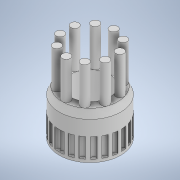
# Autodesk Inventor part: piece_roue_test_6
Saved by Autodesk Inventor 2020.1 (Build 241239000, 239)
## iProperties
Created: 2019-07-25
Part Number: piece_roue_test_6
Material: Générique
Document SubType Name: Modeling
Designer: marlo
Density: 1 g/cm^3
Appearance: Par défaut
Author: marlo
Autodesk Inventor part; units mm, degrees
ref_plane "YZ Plane" through (0, 0, 0) normal (1, 0, 0) x (0, 1, 0)
ref_plane "XZ Plane" through (0, 0, 0) normal (0, 1, 0) x (-1, 0, 0)
ref_plane "XY Plane" through (0, 0, 0) normal (0, 0, 1) x (1, 0, 0)
sketch "Esquisse2" plane through (0, 0, 0) normal (0, 1, 0) x (-1, 0, 0)
  circle A0 centre (0, 0) radius 18.5
  circle A1 centre (0, 0) radius 13.1
  dimension "d0" = 37
  dimension "d1" = 26.2
  constraints: 2 centre point, 2 coincident
  measures "d0" diameter of A0
  measures "d1" diameter of A1
extrude "Extrusion1" add sketch "Esquisse2" against normal blind 13
sketch "Esquisse3" plane through (0, 0, 0) normal (0, 1, 0) x (1, 0, 0)
  circle A0 centre (0, -15.8) radius 2.7
  line L0 (-22, 0) -> (25, 0) construction
  line L1 (-20, -18.5) -> (14, -18.5) construction
  circle A1 centre (0, 0) radius 18.5 construction
  circle A2 centre (-15.0267, 4.8825) radius 2.7
  line L2 (0, -15.8) -> (0, 0) construction
  line L3 (-15.0267, 4.8825) -> (0, 0) construction
  circle A3 centre (-15.0267, -4.8825) radius 2.7
  line L4 (0, 0) -> (-15.0267, -4.8825) construction
  line L5 (-15.0267, -4.8825) -> (-15.0267, 4.8825) construction
  line L6 (0, -31) -> (0, 24) construction
  line L7 (-15.0267, -4.8825) -> (-15.0267, -7.5825) construction
  line L8 (-15.0267, 4.8825) -> (-16.4693, 2.6002) construction
  line L9 (0, -15.8) -> (-2.3383, -17.15) construction
  circle A4 centre (-9.287, 12.7825) radius 2.7
  line L10 (0, 0) -> (-9.287, 12.7825) construction
  line L11 (-9.287, 12.7825) -> (-15.0267, 4.8825) construction
  line L12 (-9.287, 12.7825) -> (-7.7, 14.9668) construction
  circle A5 centre (-9.287, -12.7825) radius 2.7
  line L13 (-9.287, -12.7825) -> (0, 0) construction
  line L14 (-9.287, -12.7825) -> (0, -15.8) construction
  line L15 (-9.287, -12.7825) -> (-11.2119, -10.8891) construction
  line L16 (-9.287, -12.7825) -> (-15.0267, -4.8825) construction
  circle A6 centre (0, 15.8) radius 2.7
  line L17 (0, 15.8) -> (-1.5986, 17.9759) construction
  line L18 (0, 15.8) -> (0, 0) construction
  line L19 (0, 15.8) -> (-9.287, 12.7825) construction
  circle A7 centre (15.0267, 4.8825) radius 2.7
  circle A8 centre (15.0267, -4.8825) radius 2.7
  circle A9 centre (9.287, 12.7825) radius 2.7
  circle A10 centre (9.287, -12.7825) radius 2.7
  dimension "d4" = 5.4
  constraints: 40 end point, 14 equal length, 4 centre point, 4 symmetric about line, 3 horizontal, 3 point on line, 3 vertical, 1 coincident, 1 tangent, 1 vertical alignment, 21 other
extrude "Extrusion2" add sketch "Esquisse3" along normal blind 25
sketch "Esquisse4" plane through (0, -13, 0) normal (0, -1, 0) x (1, 0, 0)
  circle A0 centre (0, 0) radius 20.5
  circle A1 centre (0, 0) radius 13.1 projected
  circle A2 centre (0, 0) radius 18.5 projected
  circle A3 centre (0, 0) radius 13.1
  dimension "d9" = 2
  constraints: 2 centre point, 2 concentric, 1 coincident
  measures "d9" radial gap between concentric circles of A2 A0
extrude "Extrusion3" add sketch "Esquisse4" along normal blind 15 contours A0 | A2
sketch "Esquisse6" plane through (0, -13, 0) normal (0, 1, 0) x (1, 0, 0)
  line L0 (-3.2, -20.2487) -> (-3.1052, -19.6487)
  line L1 (0, -20.5) -> (0, -19.8926)
  arc A0 (0, -19.8926) -> (-3.1052, -19.6487) centre (-1.5707, -20.0012) ccw
  arc A1 (-3.2, -20.2487) -> (0, -20.5) centre (0, 0) ccw
  circle A2 centre (0, 0) radius 20.5 projected
  line L2 (0, 0) -> (-5.8325, -27.1444)
  line L3 (-5.4, -19.776) -> (-5.24, -19.19)
  line L4 (-8.4208, -18.6906) -> (-8.1713, -18.1368)
  arc A3 (-5.24, -19.19) -> (-8.1713, -18.1368) centre (-6.7838, -18.8811) ccw
  arc A4 (-8.4208, -18.6906) -> (-5.4, -19.776) centre (0, 0) ccw
  line L5 (0, 0) -> (0, -49) construction
  line L6 (-5.4, -19.776) -> (-3.2, -20.2487) construction
  line L7 (0, 0) -> (-12.1264, -23.3948)
  line L8 (-14.7012, -14.2872) -> (-14.2656, -13.8638)
  line L9 (-16.7512, -11.8172) -> (-16.2549, -11.4671)
  arc A5 (-14.2656, -13.8638) -> (-16.2549, -11.4671) centre (-15.4382, -12.8132) ccw
  arc A6 (-16.7512, -11.8172) -> (-14.7012, -14.2872) centre (0, 0) ccw
  line L10 (-13.0468, -15.8124) -> (-12.6602, -15.3438)
  line L11 (-10.4186, -17.6551) -> (-10.1099, -17.132)
  arc A7 (-10.1099, -17.132) -> (-12.6602, -15.3438) centre (-11.5178, -16.4273) ccw
  arc A8 (-13.0468, -15.8124) -> (-10.4186, -17.6551) centre (0, 0) ccw
  line L12 (-10.4186, -17.6551) -> (-8.4208, -18.6906) construction
  line L13 (0, 0) -> (-31.7535, -19.8843)
  line L14 (-19.6137, 5.9626) -> (-19.0325, 5.7859)
  line L15 (-18.4425, 8.9512) -> (-17.896, 8.6859)
  arc A9 (-19.0325, 5.7859) -> (-17.896, 8.6859) centre (-18.6796, 7.3203) ccw
  arc A10 (-18.4425, 8.9512) -> (-19.6137, 5.9626) centre (0, 0) ccw
  line L16 (-20.149, 3.777) -> (-19.552, 3.6651)
  line L17 (-20.4916, 0.5855) -> (-19.8844, 0.5681)
  arc A11 (-19.8844, 0.5681) -> (-19.552, 3.6651) centre (-19.9482, 2.1413) ccw
  arc A12 (-20.149, 3.777) -> (-20.4916, 0.5855) centre (0, 0) ccw
  line L18 (-20.149, 3.777) -> (-19.6137, 5.9626) construction
  line L19 (-19.2724, -6.9874) -> (-18.7014, -6.7803)
  line L20 (-17.9455, -9.9101) -> (-17.4137, -9.6164)
  line L21 (-19.9222, -4.833) -> (-19.3318, -4.6898)
  arc A13 (-17.4137, -9.6164) -> (-18.7014, -6.7803) centre (-18.2682, -8.294) ccw
  arc A14 (-19.2724, -6.9874) -> (-17.9455, -9.9101) centre (0, 0) ccw
  arc A15 (-19.3318, -4.6898) -> (-19.8269, -1.6146) centre (-19.8077, -3.189) ccw
  line L22 (-20.4324, -1.6639) -> (-19.8269, -1.6146)
  arc A16 (-20.4324, -1.6639) -> (-19.9222, -4.833) centre (0, 0) ccw
  line L23 (-20.4324, -1.6639) -> (-20.4916, 0.5855) construction
  line L24 (-17.9455, -9.9101) -> (-16.7512, -11.8172) construction
  line L25 (0, 0) -> (-31.0446, 17.2338)
  line L26 (15.493, 13.4245) -> (15.0339, 13.0267)
  line L27 (17.3986, 10.8415) -> (16.8831, 10.5202)
  arc A17 (15.0339, 13.0267) -> (16.8831, 10.5202) centre (16.1446, 11.9108) ccw
  arc A18 (17.3986, 10.8415) -> (15.493, 13.4245) centre (0, 0) ccw
  line L28 (13.9284, 15.0416) -> (13.5156, 14.5959)
  line L29 (11.4096, 17.0314) -> (11.0716, 16.5268)
  arc A19 (11.0716, 16.5268) -> (13.5156, 14.5959) centre (12.437, 15.7429) ccw
  arc A20 (13.9284, 15.0416) -> (11.4096, 17.0314) centre (0, 0) ccw
  line L30 (13.9284, 15.0416) -> (15.493, 13.4245) construction
  line L31 (4.3509, 20.033) -> (4.222, 19.4393)
  line L32 (1.1705, 20.4666) -> (1.1358, 19.8601)
  line L33 (6.5204, 19.4354) -> (6.3272, 18.8595)
  arc A21 (1.1358, 19.8601) -> (4.222, 19.4393) centre (2.7102, 19.8789) ccw
  arc A22 (4.3509, 20.033) -> (1.1705, 20.4666) centre (0, 0) ccw
  arc A23 (6.3272, 18.8595) -> (9.1935, 17.6407) centre (7.8508, 18.463) ccw
  line L34 (9.4743, 18.1793) -> (9.1935, 17.6407)
  arc A24 (9.4743, 18.1793) -> (6.5204, 19.4354) centre (0, 0) ccw
  line L35 (9.4743, 18.1793) -> (11.4096, 17.0314) construction
  line L36 (-15.4333, 13.4931) -> (-14.976, 13.0932)
  line L37 (-17.3504, 10.9186) -> (-16.8362, 10.595)
  arc A25 (-16.8362, 10.595) -> (-14.976, 13.0932) centre (-16.0916, 11.9823) ccw
  arc A26 (-15.4333, 13.4931) -> (-17.3504, 10.9186) centre (0, 0) ccw
  line L38 (-4.262, 20.0521) -> (-4.1357, 19.4579)
  arc A27 (-4.1357, 19.4579) -> (-1.0477, 19.8649) centre (-2.6219, 19.8907) ccw
  arc A28 (-1.0797, 20.4715) -> (-4.262, 20.0521) centre (0, 0) ccw
  line L39 (-1.0797, 20.4715) -> (-1.0477, 19.8649)
  line L40 (-13.8615, 15.1033) -> (-13.4507, 14.6558)
  line L41 (-11.334, 17.0819) -> (-10.9981, 16.5757)
  line L42 (-6.4341, 19.4641) -> (-6.2434, 18.8874)
  arc A29 (-6.4341, 19.4641) -> (-9.3935, 18.2212) centre (0, 0) ccw
  arc A30 (-9.1152, 17.6813) -> (-6.2434, 18.8874) centre (-7.7689, 18.4976) ccw
  line L43 (-9.3935, 18.2212) -> (-9.1152, 17.6813)
  line L44 (-9.3935, 18.2212) -> (-11.334, 17.0819) construction
  arc A31 (-11.334, 17.0819) -> (-13.8615, 15.1033) centre (0, 0) ccw
  arc A32 (-13.4507, 14.6558) -> (-10.9981, 16.5757) centre (-12.367, 15.7979) ccw
  line L45 (-13.8615, 15.1033) -> (-15.4333, 13.4931) construction
  line L46 (-1.0797, 20.4715) -> (1.1705, 20.4666) construction
  line L47 (-17.3504, 10.9186) -> (-18.4425, 8.9512) construction
  line L48 (0, 0) -> (30.2232, 16.6029)
  line L49 (20.4248, -1.7546) -> (20.494, 0.4946) construction
  arc A33 (19.8196, -1.7026) -> (19.3108, -4.7755) centre (19.7934, -3.2768) ccw
  arc A34 (19.9005, -4.9213) -> (20.4248, -1.7546) centre (0, 0) ccw
  line L50 (19.9005, -4.9213) -> (19.3108, -4.7755)
  line L51 (19.2412, -7.0728) -> (18.6711, -6.8632)
  line L52 (20.4248, -1.7546) -> (19.8196, -1.7026)
  line L53 (20.494, 0.4946) -> (19.8868, 0.4799)
  arc A35 (20.494, 0.4946) -> (20.1656, 3.6876) centre (0, 0) ccw
  arc A36 (19.5681, 3.5783) -> (19.8868, 0.4799) centre (19.9575, 2.0528) ccw
  line L54 (19.64, 5.8755) -> (19.058, 5.7014)
  line L55 (18.4821, 8.8693) -> (17.9344, 8.6065)
  line L56 (16.6986, -11.8914) -> (17.9013, -9.9896) construction
  arc A37 (18.6711, -6.8632) -> (17.3709, -9.6936) centre (18.2312, -8.375) ccw
  line L57 (20.1656, 3.6876) -> (19.5681, 3.5783)
  arc A38 (16.2038, -11.5391) -> (14.204, -13.927) centre (15.3812, -12.8815) ccw
  arc A39 (14.6377, -14.3523) -> (16.6986, -11.8914) centre (0, 0) ccw
  arc A40 (17.9013, -9.9896) -> (19.2412, -7.0728) centre (0, 0) ccw
  line L58 (16.6986, -11.8914) -> (16.2038, -11.5391)
  line L59 (14.6377, -14.3523) -> (14.204, -13.927)
  line L60 (17.9013, -9.9896) -> (17.3709, -9.6936)
  arc A41 (17.9344, 8.6065) -> (19.058, 5.7014) centre (18.7119, 7.2374) ccw
  arc A42 (19.64, 5.8755) -> (18.4821, 8.8693) centre (0, 0) ccw
  arc A43 (5.3122, -19.7998) -> (8.3378, -18.7278) centre (0, 0) ccw
  arc A44 (8.0907, -18.1729) -> (5.1548, -19.2131) centre (6.7, -18.911) ccw
  line L61 (5.3122, -19.7998) -> (5.1548, -19.2131)
  line L62 (20.1656, 3.6876) -> (19.64, 5.8755) construction
  line L63 (10.3401, -17.7012) -> (10.0337, -17.1767)
  arc A45 (12.592, -15.3999) -> (10.0337, -17.1767) centre (11.4448, -16.4782) ccw
  line L64 (12.9765, -15.8701) -> (12.592, -15.3999)
  arc A46 (10.3401, -17.7012) -> (12.9765, -15.8701) centre (0, 0) ccw
  line L65 (8.3378, -18.7278) -> (8.0907, -18.1729)
  line L66 (17.3986, 10.8415) -> (18.4821, 8.8693) construction
  line L67 (0, 0) -> (5.8388, -27.7733)
  line L68 (3.1101, -20.2627) -> (3.018, -19.6623)
  arc A47 (3.018, -19.6623) -> (-0.0883, -19.8924) centre (1.4819, -20.008) ccw
  arc A48 (-0.0909, -20.4998) -> (3.1101, -20.2627) centre (0, 0) ccw
  line L69 (-0.0909, -20.4998) -> (-0.0883, -19.8924)
  line L70 (3.1101, -20.2627) -> (5.3122, -19.7998) construction
  circle A49 centre (0, 0) radius 20.5
  point P0 (0, -18.5)
  point P1 (-10.874, -14.9668)
  point P2 (-7.5992, -16.8672)
  point P3 (-15.117, -10.6643)
  point P4 (-9.4021, -15.9327)
  point P5 (-16.6432, 8.0779)
  point P6 (-18.2127, -3.2475)
  point P7 (-18.4925, 0.5284)
  point P8 (-16.1947, -8.9432)
  point P9 (-18.439, -1.5016)
  point P10 (15.7012, 9.7838)
  point P11 (6.9518, 17.1442)
  point P12 (10.2965, 15.3698)
  point P13 (1.0563, 18.4698)
  point P14 (8.5499, 16.4058)
  point P15 (-15.6576, 9.8533)
  point P16 (-6.8756, 17.1748)
  point P17 (-0.9744, 18.4743)
  point P18 (-10.2282, 15.4154)
  point P19 (-8.4771, 16.4435)
  point P20 (18.4321, -1.5834)
  point P21 (18.1981, -3.3283)
  point P22 (18.4946, 0.4463)
  point P23 (16.6789, 8.004)
  point P24 (16.1549, -9.015)
  point P25 (15.0695, -10.7313)
  point P26 (7.5243, -16.9007)
  point P27 (9.3313, -15.9742)
  point P28 (10.8075, -15.0149)
  point P29 (-0.0821, -18.4998)
  point P30 (-0.0435, -19.6183)
  point P31 (20.494, 0.4946)
  dimension "d17" = 3.2
  dimension "d34" = 0.6
  dimension "d35" = 1.5744
  dimension "d36" = 2.2
  constraints: 144 symmetric about line, 142 end point, 97 point on circle, 49 centre point, 6 equal length, 2 coincident, 2 line through centre, 1 vertical, 46 other
  measures "d17" horizontal distance of L1.start L0.start
  measures "d34" vertical distance of L0.start L0.end
  measures "d35" radius of A0
  measures "d36" horizontal distance of L3.start L0.start
extrude "Extrusion5" cut sketch "Esquisse6" against normal blind 15 contours L0 A0 A47 L69 A1 | L69 A47 A0 L1 A1 | A47 L68 A2 L1 A0 | A2 L4 A3 L3 | A2 L10 A7 L11 | A2 L19 A13 L20 | L9 A5 L8 A2 | A2 L36 A25 L37 | L15 A9 L14 A2 | A2 L54 A41 L55 | L27 A17 L26 A2 | L61 A44 L65 A2 | A2 L22 A15 L21 | L16 A11 L17 A2 | A2 L53 A36 L57 | L28 A19 L29 A2 | L63 A45 L64 A2 | A2 L42 A30 L43 | L34 A23 L33 A2 | L59 A38 L58 A2 | A2 L50 A33 L52 | A2 L39 A27 L38 | L31 A21 L32 A2 | L60 A37 L51 A2
sketch "Esquisse7" plane through (0, -28, 0) normal (0, -1, 0) x (1, 0, 0)
  arc A0 (19.64, -5.8755) -> (20.4248, 1.7546) centre (0, 0) ccw projected
  circle A1 centre (0, 0) radius 20.5
  circle A2 centre (0, 0) radius 13.1
  point P0 (15.8414, 13.0116)
  point P1 (14.4826, 14.5088)
  point P2 (20.5, 0)
  point P3 (-3.2, 20.2487)
  point P4 (0, 20.5)
  point P5 (20.494, -0.4946)
  point P6 (20.4248, 1.7546)
  point P7 (20.5, 0)
  constraints: 2 centre point, 2 coincident, 1 point on circle
extrude "Extrusion6" add sketch "Esquisse7" along normal blind 2
sketch "Esquisse8" plane through (0, 0, 0) normal (0, 1, 0) x (1, 0, 0)
  arc A0 (-8.887, -16.2257) -> (-7.0807, -17.0913) centre (0, 0) ccw projected
  circle A1 centre (0, 0) radius 18.5
  arc A2 (19.9005, -4.9213) -> (20.4248, -1.7546) centre (0, 0) ccw projected
  circle A3 centre (0, 0) radius 20.5
  point P0 (-7.8462, -18.939)
  point P1 (-9.6565, -18.0832)
  point P2 (-8.887, -16.2257)
  point P3 (-7.8462, -18.939)
  point P4 (-9.6565, -18.0832)
  point P5 (-3.2, -20.2487)
  point P6 (0, -20.5)
  constraints: 2 coincident, 1 centre point, 3 other
extrude "Extrusion7" add sketch "Esquisse8" against normal blind 15
chamfer "Chanfrein2" distance 2 distance2 5 2 edges at (-20.2247, 0, -3.3482) (20.2247, 0, 3.3482) measured on face at (19.7314, 0, 3.2666) measured on face at (-19.7314, 0, -3.2666)
